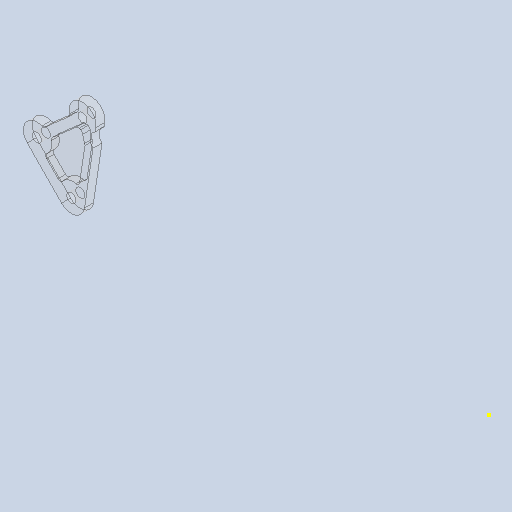
# Autodesk Inventor part: アーム ツインアーム先端押さえ
Saved by Autodesk Inventor 2023 (Build 270158030, 158C)
## iProperties
Created: 2020-05-03
Part Number: アーム ツインアーム先端押さえ
Material: ポリカーボネート、クリア
Document SubType Name: Modeling
Designer: mozar
Density: 1.2 g/cm^3
Appearance: ポリカーボネート - クリア
Mass: 1.14014 g
Surface Area: 13.7283 cm^2
Volume: 0.950116 cm^3
Author: mozar
Autodesk Inventor part; units mm, degrees
ref_plane "YZ Plane" through (0, 0, 0) normal (1, 0, 0) x (0, 1, 0)
ref_plane "XZ Plane" through (0, 0, 0) normal (0, 1, 0) x (-1, 0, 0)
ref_plane "XY Plane" through (0, 0, 0) normal (0, 0, 1) x (1, 0, 0)
sketch "スケッチ1" plane through (0, 0, 0) normal (0, 0, 1) x (1, 0, 0)
  circle A0 centre (-84.1159, 33.5789) radius 1.5
  circle A1 centre (-105.2485, 37.922) radius 1.5
  circle A2 centre (-132.6852, 21.2646) radius 1.5
  circle A3 centre (-77.8119, 54.5794) radius 1.5
  circle A4 centre (-112.1063, 12.5661) radius 1.5
  circle A5 centre (-60.4494, 64.5064) radius 1.5
  circle A6 centre (-64.4423, 49.0046) radius 1.5
  circle A7 centre (-44.4492, 64.0137) radius 1.5
  line L0 (-44.233, 71.0354) -> (-60.2332, 71.5281)
  arc A8 (-60.2332, 71.5281) -> (-64.0951, 70.5113) centre (-60.4494, 64.5064) ccw
  line L1 (-64.0951, 70.5113) -> (-153.1544, 16.4415)
  arc A9 (-153.1544, 16.4415) -> (-154.1888, 0.0236) centre (-147.9517, 7.8722) ccw
  line L2 (-154.1888, 0.0236) -> (-141.4408, -10.1069)
  arc A10 (-141.4408, -10.1069) -> (-131.6607, -10.2415) centre (-136.4636, -3.8437) ccw
  arc A11 (-40.2316, 58.3956) -> (-44.233, 71.0354) centre (-44.4492, 64.0137) ccw
  circle A12 centre (-147.9517, 7.8722) radius 1.5
  circle A13 centre (-136.4636, -3.8437) radius 1.5
  circle A14 centre (-132.6852, 21.2646) radius 1.5
  circle A15 centre (-132.6852, 21.2646) radius 4.5
  circle A16 centre (-147.9517, 7.8722) radius 4.5
  circle A17 centre (-136.4636, -3.8437) radius 1.5
  circle A18 centre (-136.4636, -3.8437) radius 4.5
  line L3 (-151.1648, 4.7216) -> (-139.6766, -6.9943)
  line L4 (-132.0137, -4.5133) -> (-128.2279, 20.6438)
  line L5 (-135.6527, 24.6475) -> (-150.9193, 11.255)
  circle A19 centre (-112.1063, 12.5661) radius 4.5
  point P0 (0, 0)
  point P1 (0, 0)
  point P2 (-128.2353, 20.595)
  dimension "d0" = 9
  dimension "d1" = 9
  dimension "d2" = 9
  dimension "d5" = 9
  constraints: 19 centre point, 12 end point, 12 point on circle, 7 coincident, 4 tangent, 11 other
  measures "d1" diameter of A16
  measures "d2" diameter of A18
  measures "d5" diameter of A19
extrude "押し出し1" add sketch "スケッチ1" against normal blind 3 contours A15 L4 A18 L3 A16 L5 | A16 | A18
sketch "スケッチ2" plane through (0, 0, 0) normal (0, 0, 1) x (1, 0, 0)
  circle A0 centre (-142.0156, -13.6386) radius 1.5
  line L0 (-193.8461, -47.1997) -> (-168.4977, -27.8921)
  arc A1 (-162.0848, -31.6046) -> (-168.4977, -27.8921) centre (-166.0653, -31.0855) ccw
  line L1 (-162.0848, -31.6046) -> (-161.5284, -29.669)
  arc A2 (-161.365, -29.2693) -> (-161.5284, -29.669) centre (-159.6062, -30.2215) ccw
  line L2 (-161.365, -29.2693) -> (-154.7883, -17.1215)
  arc A3 (-151.2707, -19.0259) -> (-154.7883, -17.1215) centre (-153.0295, -18.0737) ccw
  line L3 (-151.2707, -19.0259) -> (-154.509, -25.0074)
  arc A4 (-154.509, -25.0074) -> (-153.0293, -26.2832) centre (-153.6296, -25.4835) ccw
  line L4 (-153.0293, -26.2832) -> (-128.1569, -7.6112)
  arc A5 (-128.1569, -7.6112) -> (-126.988, -5.6349) centre (-129.958, -5.212) ccw
  line L5 (-126.988, -5.6349) -> (-123.9066, 16.0052)
  arc A6 (-123.9066, 16.0052) -> (-127.0915, 19.4204) centre (-126.8767, 16.4281) ccw
  line L6 (-127.0915, 19.4204) -> (-130.5344, 19.1732)
  arc A7 (-134.5152, 18.8875) -> (-130.5344, 19.1732) centre (-132.6852, 21.2646) ccw
  line L7 (-134.5152, 18.8875) -> (-148.6695, 17.8715)
  arc A8 (-148.6695, 17.8715) -> (-157.1727, 11.806) centre (-147.9517, 7.8722) ccw
  line L8 (-157.1727, 11.806) -> (-166.1369, -9.2063)
  line L9 (-166.1369, -9.2063) -> (-193.8461, -47.1997)
  circle A9 centre (-126.8767, 16.4281) radius 1.5
  circle A10 centre (-158.5928, -9.2025) radius 1.5
  arc A11 (-128.5265, 10.8915) -> (-134.9494, 9.8931) centre (-131.7379, 10.3923) ccw
  arc A12 (-133.9759, -5.9529) -> (-128.5265, 10.8915) centre (-147.9517, 7.8722) ccw
  arc A13 (-138.597, -1.3817) -> (-133.9759, -5.9529) centre (-136.2864, -3.6673) ccw
  arc A14 (-138.597, -1.3817) -> (-134.9494, 9.8931) centre (-147.9517, 7.8722) ccw
  circle A15 centre (-147.9517, 7.8722) radius 4.025
  arc A16 (-150.9193, 11.255) -> (-151.1648, 4.7216) centre (-147.9517, 7.8722) ccw projected
  line L10 (-151.1648, 4.7216) -> (-139.6766, -6.9943) projected
  arc A17 (-139.6766, -6.9943) -> (-132.0137, -4.5133) centre (-136.4636, -3.8437) ccw projected
  line L11 (-132.0137, -4.5133) -> (-128.2353, 20.595) projected
  arc A18 (-128.2353, 20.595) -> (-135.6527, 24.6475) centre (-132.6852, 21.2646) ccw projected
  line L12 (-135.6527, 24.6475) -> (-150.9193, 11.255) projected
  circle A19 centre (-132.6852, 21.2646) radius 1.5 projected
  circle A20 centre (-147.9517, 7.8722) radius 1.5 projected
  circle A21 centre (-136.4636, -3.8437) radius 1.5 projected
  circle A22 centre (-126.8767, 16.4281) radius 3.25
  point P0 (0, 0)
  point P1 (0, 0)
  dimension "d6" = 6.5
  constraints: 24 point on circle, 20 end point, 17 centre point, 1 coincident, 84 other
  measures "d6" diameter of A22
extrude "押し出し2" cut sketch "スケッチ2" against normal blind 10 contours A22 L5 A6 L6 | L6 A6 L5 A22 L11 | L11 A22 | A9
sketch "スケッチ3" plane through (0, 0, -3) normal (0, 0, -1) x (-1, 0, 0)
  arc A0 (129.2038, 14.1593) -> (128.433, 19.2812) centre (126.8767, 16.4281) ccw projected
  line L0 (129.2038, 14.1593) -> (132.0137, -4.5133) projected
  arc A1 (132.0137, -4.5133) -> (139.6766, -6.9943) centre (136.4636, -3.8437) ccw projected
  line L1 (139.6766, -6.9943) -> (151.1648, 4.7216) projected
  arc A2 (151.1648, 4.7216) -> (150.9193, 11.255) centre (147.9517, 7.8722) ccw projected
  line L2 (150.9193, 11.255) -> (135.6527, 24.6475) projected
  arc A3 (135.6527, 24.6475) -> (128.2353, 20.595) centre (132.6852, 21.2646) ccw projected
  line L3 (128.2353, 20.595) -> (128.433, 19.2812) projected
  circle A4 centre (132.6852, 21.2646) radius 1.5 projected
  circle A5 centre (147.9517, 7.8722) radius 1.5 projected
  circle A6 centre (136.4636, -3.8437) radius 1.5 projected
  line L4 (149.0228, 6.822) -> (137.5346, -4.8939)
  arc A7 (134.9803, -4.0669) -> (137.5346, -4.8939) centre (136.4636, -3.8437) ccw
  line L5 (134.9803, -4.0669) -> (132.3502, 13.4109)
  arc A8 (132.3502, 13.4109) -> (131.2198, 20.9225) centre (126.8767, 16.4281) ccw
  line L6 (131.2198, 20.9225) -> (131.2019, 21.0414)
  arc A9 (133.6744, 22.3923) -> (131.2019, 21.0414) centre (132.6852, 21.2646) ccw
  line L7 (133.6744, 22.3923) -> (148.9409, 8.9998)
  arc A10 (149.0228, 6.822) -> (148.9409, 8.9998) centre (147.9517, 7.8722) ccw
  circle A11 centre (132.6852, 21.2646) radius 1.5 projected
  circle A12 centre (132.6852, 21.2646) radius 4.5
  circle A13 centre (147.9517, 7.8722) radius 4.5
  circle A14 centre (136.4636, -3.8437) radius 1.5 projected
  circle A15 centre (136.4636, -3.8437) radius 4.5
  point P0 (0, 0)
  point P1 (134.349, 0.1285)
  point P2 (140.505, -1.8646)
  point P3 (146.0523, 3.7927)
  point P4 (145.7516, 11.7976)
  point P5 (136.8637, 19.5944)
  point P6 (133.1164, 16.7854)
  dimension "d9" = 3
  constraints: 8 end point, 8 point on circle, 4 centre point, 3 coincident, 16 other
  measures "d9" distance between parallel lines of L1 L4
extrude "押し出し3" cut sketch "スケッチ3" against normal blind 2.5 contours A12 L7 A13 L4 A15 L5 A8
sketch "スケッチ4" plane through (0, 0, -3) normal (0, 0, -1) x (-1, 0, 0)
  line L0 (140.505, -1.8646) -> (146.0523, 3.7927) projected
  arc A0 (145.7516, 11.7976) -> (146.0523, 3.7927) centre (147.9517, 7.8722) ccw projected
  line L1 (145.7516, 11.7976) -> (136.8637, 19.5944) projected
  arc A1 (133.1164, 16.7854) -> (136.8637, 19.5944) centre (132.6852, 21.2646) ccw projected
  arc A2 (132.3502, 13.4109) -> (133.1164, 16.7854) centre (126.8767, 16.4281) ccw projected
  line L2 (132.3502, 13.4109) -> (134.349, 0.1285) projected
  arc A3 (140.505, -1.8646) -> (134.349, 0.1285) centre (136.4636, -3.8437) ccw projected
  circle A4 centre (136.4636, -3.8437) radius 1.5 projected
  circle A5 centre (147.9517, 7.8722) radius 1.5 projected
  circle A6 centre (132.6852, 21.2646) radius 1.5 projected
  line L3 (151.1648, 4.7216) -> (139.6766, -6.9943) projected
  arc A7 (132.0137, -4.5133) -> (139.6766, -6.9943) centre (136.4636, -3.8437) ccw projected
  line L4 (132.0137, -4.5133) -> (129.2038, 14.1593) projected
  arc A8 (129.2038, 14.1593) -> (128.433, 19.2812) centre (126.8767, 16.4281) ccw projected
  line L5 (128.433, 19.2812) -> (128.2353, 20.595) projected
  arc A9 (135.6527, 24.6475) -> (128.2353, 20.595) centre (132.6852, 21.2646) ccw projected
  line L6 (135.6527, 24.6475) -> (150.9193, 11.255) projected
  arc A10 (151.1648, 4.7216) -> (150.9193, 11.255) centre (147.9517, 7.8722) ccw projected
  line L7 (147.9517, 7.8722) -> (132.6852, 21.2646) construction
  line L8 (148.9409, 8.9998) -> (133.6744, 22.3923)
  line L9 (131.696, 20.137) -> (146.9626, 6.7446)
  arc A11 (146.9626, 6.7446) -> (148.9409, 8.9998) centre (147.9517, 7.8722) ccw
  arc A12 (133.6744, 22.3923) -> (131.696, 20.137) centre (132.6852, 21.2646) ccw
  circle A13 centre (132.6852, 21.2646) radius 4.5
  circle A14 centre (147.9517, 7.8722) radius 4.5
  point P0 (0, 0)
  point P1 (140.3185, 14.5684)
  point P2 (145.7516, 11.7976)
  point P3 (135.6527, 24.6475)
  point P4 (134.8854, 17.3392)
  point P5 (143.7732, 9.5424)
  dimension "d12" = 3
  constraints: 8 end point, 4 point on circle, 4 tangent, 2 centre point, 2 coincident, 1 concentric, 1 midpoint, 1 parallel, 6 other
  measures "d12" diameter of A12
extrude "押し出し4" cut sketch "スケッチ4" against normal blind 10 contours L1 A13 L6 A14
extrude "押し出し5" add sketch "スケッチ4" against normal blind 3 contours L9 A1 L1 A0
sketch "スケッチ5" plane through (0, 0, -3) normal (0, 0, -1) x (-1, 0, 0)
  point P0 (0, 0)
fillet "フィレット1" radius 1 7 edges at (-134.8854, 17.3392, -1.75) (-133.1164, 16.7854, -1.75) (-132.3502, 13.4109, -1.75) (-143.7732, 9.5424, -1.75) (-146.0523, 3.7927, -1.75) (-140.505, -1.8646, -1.75) (-134.349, 0.1285, -1.75)
fillet "フィレット2" radius 1 2 edges at (-136.8637, 19.5944, -1.5) (-145.7516, 11.7976, -1.5)
